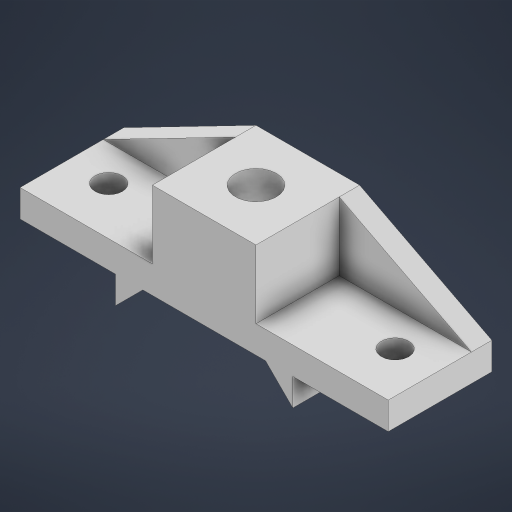
# Autodesk Inventor part: Part2
Saved by Autodesk Inventor 2024 (Build 280153000, 153)
## iProperties
Created: 2024-02-24
Part Number: Part2
Material: Generic
Document SubType Name: Modeling
Designer: Papryk
Density: 1 g/cm^3
Appearance: Default
Author: Papryk
Autodesk Inventor part; units mm, degrees
ref_plane "YZ Plane" through (0, 0, 0) normal (1, 0, 0) x (0, 1, 0)
ref_plane "XZ Plane" through (0, 0, 0) normal (0, 1, 0) x (-1, 0, 0)
ref_plane "XY Plane" through (0, 0, 0) normal (0, 0, 1) x (1, 0, 0)
sketch "Sketch1" plane through (0, 0, 0) normal (0, 0, 1) x (1, 0, 0)
  line L0 (0, 29.8421) -> (-38, 29.8421)
  line L1 (-38, 29.8421) -> (-38, -20.1579)
  line L2 (-38, -40.1579) -> (0, -40.1579)
  line L3 (0, -40.1579) -> (0, 29.8421)
  line L4 (-135, -40.1579) -> (-135, -20.1579)
  line L5 (-135, -20.1579) -> (-38, -20.1579)
  line L6 (0, -20.1579) -> (0, -40.1579)
  line L7 (-65, -60.1579) -> (-65, -40.1579)
  line L8 (-65, -60.1579) -> (-45, -40.1579)
  line L9 (0, -40.1579) -> (-45, -40.1579)
  line L10 (-65, -40.1579) -> (-135, -40.1579)
  line L11 (-135, -20.1579) -> (-38, 29.8421)
  point P0 (0, 0)
  dimension "d17" = 20
  constraints: 24 end point, 5 parallel, 3 horizontal, 3 perpendicular
  measures "d17" distance of L4.start L4.end
extrude "Extrusion1" add sketch "Sketch1" along normal blind 15 contours L1 L5 L11
extrude "Extrusion2" add sketch "Sketch1" along normal blind 76 contours L3 L2 L9 L8 L7 L10 L4 L5 L1 L0
sketch "Sketch2" plane through (-38, 29.8421, 0) normal (0, 1, 0) x (1, 0, 0)
  circle A0 centre (-67, -41) radius 10
  circle A1 centre (38, -38) radius 15
  dimension "d31" = 20
  dimension "d34" = 30
  constraints: 2 centre point
  measures "d31" diameter of A0
  measures "d34" diameter of A1
extrude "Extrusion3" cut sketch "Sketch2" against normal through all contours A0
extrude "Extrusion4" cut sketch "Sketch2" against normal through all contours A1
mirror "Mirror1" about plane through (0, 0, 0) normal (1, 0, 0)
body "Solid1"
